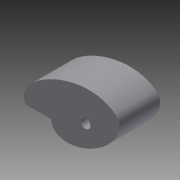
# Autodesk Inventor part: cam 3
Saved by Autodesk Inventor 2014 (Build 180170000, 170)
## iProperties
Created: 2014-05-19
Part Number: cam 3
Material: Generic
Document SubType Name: Modeling
Designer: jyesowitz
Density: 1 g/cm^3
Appearance: Default
Author: jyesowitz
Autodesk Inventor part; units mm, degrees
ref_plane "YZ Plane" through (0, 0, 0) normal (1, 0, 0) x (0, 1, 0)
ref_plane "XZ Plane" through (0, 0, 0) normal (0, 1, 0) x (-1, 0, 0)
ref_plane "XY Plane" through (0, 0, 0) normal (0, 0, 1) x (1, 0, 0)
sketch "Sketch1" plane through (0, 0, 0) normal (0, 0, 1) x (1, 0, 0)
  ellipse E0 centre (0, 0) end of major axis (40.4102, 24.5237) minor radius 24.6126 (-42.3793, -17.1629) -> (36.8507, 28.3784) ccw
  line L0 (36.8507, 28.3784) -> (-3.6148, 58.2557) construction
  line L1 (-3.6148, 58.2557) -> (-80.2799, 14.5275) construction
  line L2 (-80.2799, 14.5275) -> (-81.5178, -4.6582) construction
  line L3 (-81.5178, -4.6582) -> (-73.9291, -17.1629) construction
  spline S0 degree 4 poles (36.8507, 28.3784) (-3.6148, 58.2557) (-80.2799, 14.5275) (-81.5178, -4.6582) (-73.9291, -17.1629) knots 1 1 1 1 1 2 2 2 2 2
  line L4 (-73.9291, -17.1629) -> (-42.3793, -17.1629)
  circle A0 centre (0, 0) radius 6.35
  point P0 (-58.1542, -17.1629)
  dimension "d7" = 47.2694
  dimension "d13" = 24.6126
  dimension "d0" = 75.8952
  dimension "d2" = 50.3002
  dimension "d3" = 88.2592
  dimension "d4" = 19.2256
  dimension "d5" = 14.6272
  dimension "d6" = 45.7227
  dimension "d9" = 113.861
  dimension "d10" = 58.2557
  dimension "d14" = 12.7
  constraints: 2 coincident, 2 end point, 1 centre point, 1 horizontal, 1 midpoint, 9 other
  measures "d0" distance of L3.end point (0, 0)
  measures "d2" distance of L0.start L0.end
  measures "d3" distance of L0.end L1.end
  measures "d4" distance of L1.end L2.end
  measures "d5" distance of L2.end L3.end
  measures "d6" distance of point (0, 0) L4.end
  measures "d9" angle of L1 L0
  measures "d10" vertical distance of point (0, 0) L0.end
  measures "d14" diameter of A0
extrude "Extrusion1" add sketch "Sketch1" against normal blind 50.8
body "Solid1"
